Solenoid JF0520B (Autodesk Fusion 360 design; units mm, degrees)
Autodesk Fusion 360 part; units mm, degrees
sketch "Sketch1" plane through (0, 0, 0) normal (0, 1, 0) x (1, 0, 0)
  circle A0 centre (0, 0) radius 7
  circle A1 centre (0, 0) radius 3
  line L0 (6.5, 8) -> (-6.5, 8)
  line L1 (-6.5, 8) -> (-6.5, -8)
  line L2 (-6.5, -8) -> (6.5, -8)
  line L3 (6.5, -8) -> (6.5, 8)
  line L4 (6.5, 8) -> (-6.5, -8) construction
  line L5 (-6.5, 8) -> (6.5, -8) construction
  dimension "d3" = 14
  dimension "d6" = 6
  dimension "d9" = 13
  dimension "d10" = 16
  constraint coincident A0.centre A1.centre
  constraint horizontal L0
  constraint perpendicular L0 L1
  constraint parallel L0 L2
  constraint parallel L1 L3
  constraint coincident L4 A0.centre
  constraint coincident L5 A0.centre
  measures "d3" diameter of A0
  measures "d6" diameter of A1
  measures "d9" distance of L1.end L2.end
  measures "d10" distance of L0.end L1.end
sketch "Sketch2" plane through (0, 0, 0) normal (1, 0, 0) x (0, 1, 0)
  line L0 (0, -8) -> (20, -8)
  line L1 (20, -8) -> (20, 8)
  line L2 (20, 8) -> (0, 8)
  line L3 (0, 8) -> (0, -8)
  dimension "d4" = 20
  dimension "d5" = 16
  constraint horizontal L0
  constraint vertical L1
  constraint horizontal L2
  constraint vertical L3
  measures "d4" distance of L0.start L0.end
  measures "d5" distance of L0.start L2.end
extrude "Extrude1" add sketch "Sketch1" along normal blind 18 contours A0 L3 | A0 L1 L3 | A0 L1 makes body 1
extrude "Extrude2" add sketch "Sketch2" along normal mid plane 13 thin wall 1 inside separate body makes body 2
move_body "Move1" bodies 1 to x (1, 0, 0) y (0, 1, 0) z (0, 0, 1) at (0, 1, 0)
extrude "Extrude3" cut sketch "Sketch1" along normal blind 20 contours A1 bodies 2
extrude "Extrude4" add sketch "Sketch1" against normal blind 47 separate body contours A1 makes body 3
move_face "MoveFace1" to x (1, 0, 0) y (0, 1, 0) z (0, 0, 1) at (0, -10, 0) 1 faces at (2.9963, -31.3333, 0.1495) on bodies 3
move_face "MoveFace2" to x (1, 0, 0) y (0, 1, 0) z (0, 0, 1) at (0, -16, 0) 1 faces at (2.9963, -31.3333, 0.1495) on bodies 3
move_body "Move2" bodies 3 to x (1, 0, 0) y (0, 1, 0) z (0, 0, 1) at (0, 25, 0)
sphere "SpherePrimitive1" add diameter 8.5 placed x (-1, 0, 0) y (0, 0, 1) z (0, 1, 0) at (0, 20, 0) separate body makes body 4
move_body "Move3" bodies 4 to x (1, 0, 0) y (0, 1, 0) z (0, 0, 1) at (0, 2, 0)
delete_face "DeleteFace1" 1 faces at (4.0293, 23.0046, -0.9043) on bodies 4
